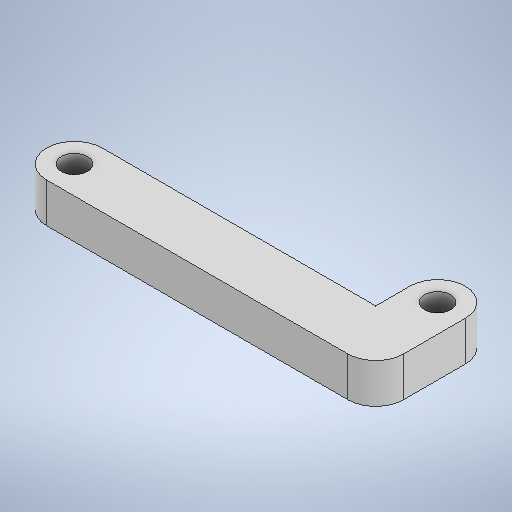
# Autodesk Inventor part: connector
Saved by Autodesk Inventor 2025.1 (Build 291241020, 241B)
## iProperties
Created: 2025-05-24
Part Number: connector
Material: Generic
Document SubType Name: Modeling
Designer: omiye
Density: 1 g/cm^3
Appearance: Default
Author: omiye
Autodesk Inventor part; units mm, degrees
ref_plane "YZ Plane" through (0, 0, 0) normal (1, 0, 0) x (0, 1, 0)
ref_plane "XZ Plane" through (0, 0, 0) normal (0, 1, 0) x (-1, 0, 0)
ref_plane "XY Plane" through (0, 0, 0) normal (0, 0, 1) x (1, 0, 0)
sketch "Sketch1" plane through (0, 0, 0) normal (0, 1, 0) x (-1, 0, 0)
  line L0 (-19, -3.5) -> (-19, 3.5)
  line L1 (-19, 3.5) -> (19, 3.5)
  line L2 (19, 3.5) -> (19, -3.5)
  line L3 (19, -3.5) -> (-19, -3.5)
  line L4 (-19, -3.5) -> (19, 3.5) construction
  line L5 (-19, 3.5) -> (19, -3.5) construction
  circle A0 centre (19, 0) radius 1.65
  line L6 (19, 3.5) -> (22.5, 3.5)
  line L7 (22.5, 3.5) -> (22.5, -3.5)
  line L8 (22.5, -3.5) -> (19, -3.5)
  line L9 (19, -3.5) -> (19, 3.5)
  line L10 (-19, 0) -> (-19, -7.8)
  line L11 (-22.5, 14.8) -> (-22.5, -7.8)
  line L12 (-22.5, -7.8) -> (-15.5, -7.8)
  line L13 (-15.5, -7.8) -> (-15.5, 14.8)
  line L14 (-15.5, 14.8) -> (-22.5, 14.8)
  line L15 (-22.5, 14.8) -> (-15.5, -7.8) construction
  line L16 (-22.5, -7.8) -> (-15.5, 14.8) construction
  line L17 (-19, 3.5) -> (-22.5, 3.5)
  circle A1 centre (-19, -7.8) radius 1.65
  line L18 (-15.5, -7.8) -> (-22.5, -7.8)
  line L19 (-22.5, -7.8) -> (-22.5, -11.3)
  line L20 (-22.5, -11.3) -> (-15.5, -11.3)
  line L21 (-15.5, -11.3) -> (-15.5, -7.8)
  point P0 (0, 0)
  point P1 (-22.5, -7.8)
  point P2 (-15.5, -3.5)
  dimension "d0" = 7
  dimension "d1" = 38
  dimension "d2" = 3.3
  dimension "d3" = 3.5
  dimension "d4" = 7.8
  dimension "d5" = 7
  dimension "d6" = 3.3
  dimension "d7" = 3.5
  constraints: 44 end point, 9 parallel, 7 midpoint, 4 perpendicular, 2 centre point, 2 horizontal, 1 coincident, 1 point on line, 1 vertical
  measures "d0" distance of L0.start L0.end
  measures "d1" distance of L0.end L1.end
  measures "d2" diameter of A0
  measures "d3" distance of L7.end L8.end
  measures "d4" distance of L10.start L10.end
  measures "d5" distance of L12.end L11.end
  measures "d6" diameter of A1
  measures "d7" distance of L19.end L18.end
extrude "Extrusion1" add sketch "Sketch1" along normal blind 5 contours L10 A1 L12 L11 L17 L0 | L0 L1 L13 L3 | L3 L13 L12 A1 L10 | L13 L1 L2 A0 L3 | L2 A0 L6 L7 L8 | L21 L20 L19 L12 A1
fillet "Fillet1" radius 3.5 5 edges at (22.5, 2.5, -11.3) (15.5, 2.5, -11.3) (22.5, 2.5, 3.5) (-22.5, 2.5, 3.5) (-22.5, 2.5, -3.5)
body "Solid1"
